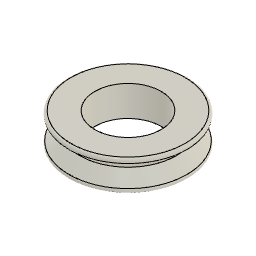
Counterweight Wheel (Autodesk Fusion 360 design; units mm, degrees)
Autodesk Fusion 360 part; units mm, degrees
sketch "Sketch1" plane through (0, 0, 0) normal (0, 0, 1) x (1, 0, 0)
  circle A0 centre (0, 0) radius 6.55
  circle A1 centre (0, 0) radius 12.5
  dimension "d1" = 13.1
  dimension "d2" = 25
  constraint coincident A0.centre A1.centre
  measures "d1" diameter of A0
  measures "d2" diameter of A1
extrude "Extrude1" add sketch "Sketch1" along normal blind 6
sketch "Sketch2" plane through (0, 0, 0) normal (0, 1, 0) x (1, 0, 0)
  line L0 (-12.5, -6) -> (12.5, -6)
  line L1 (-12.5, 0) -> (12.5, 0)
  line L2 (12.5, 0) -> (9.5, -3)
  line L3 (9.5, -3) -> (12.5, -6)
  line L4 (12.5, -6) -> (12.5, 0)
  dimension "d5" = 45
  dimension "d6" = 45
  constraint coincident L1.end L2.start
  constraint coincident L0.end L3.end
  measures "d5" angle of L1 L2
  measures "d6" angle of L0 L3
revolve "Revolve1" cut sketch "Sketch2" angle 360 about axis through (0, 0, 1.75) along (0, 0, 1)
fillet "Fillet1" radius 0.5 2 edges at (-11.6541, -4.5202, 0) (-11.6541, -4.5202, 6)
